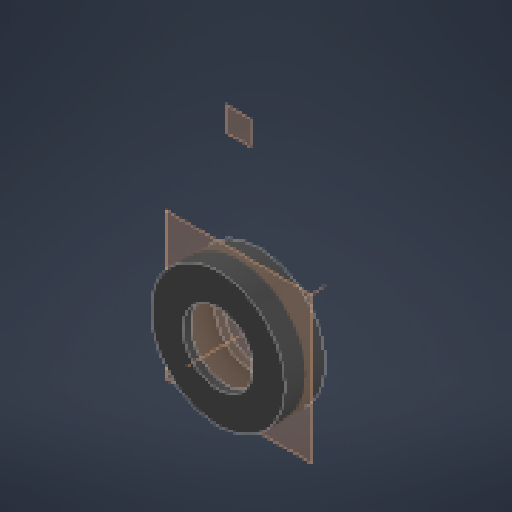
# Autodesk Inventor part: custom_bearing
Saved by Autodesk Inventor 2026.1 (Build 301233020, 233B)
## iProperties
Created: 2025-11-24
Part Number: custom_bearing
Material: 고무, 검은색
Document SubType Name: Modeling
Designer: jaewook
Density: 0.93 g/cm^3
Appearance: 고무 - 검은색
Author: jaewook
Autodesk Inventor part; units mm, degrees
ref_plane "YZ Plane" through (0, 0, 0) normal (1, 0, 0) x (0, 1, 0)
ref_plane "XZ Plane" through (0, 0, 0) normal (0, 1, 0) x (-1, 0, 0)
ref_plane "XY Plane" through (0, 0, 0) normal (0, 0, 1) x (1, 0, 0)
ref_plane "작업 평면1" through (0, -41, 8.5) normal (0, 0, 1) x (1, 0, 0)
sketch "스케치1" plane through (0, -41, 8.5) normal (0, 0, 1) x (1, 0, 0)
  circle A0 centre (0, -40.5) radius 15 projected
  circle A1 centre (0, -40.5) radius 5 projected
  circle A2 centre (0, -40.5) radius 14.8
  circle A3 centre (0, -40.5) radius 5.3
  circle A4 centre (0, -40.5) radius 13.1
  circle A5 centre (0, -40.5) radius 7
  point P0 (0, 41)
  dimension "d0" = 0.2
  dimension "d1" = 0.3
  dimension "d2" = 1.7
  dimension "d3" = 1.7
  constraints: 4 centre point
  measures "d0" radial gap between concentric circles of A0 A2
  measures "d1" radial gap between concentric circles of A1 A3
  measures "d2" radial gap between concentric circles of A3 A5
  measures "d3" radial gap between concentric circles of A2 A4
extrude "돌출1" add sketch "스케치1" along normal mid plane 9 contours A2
ref_plane "작업 평면2" through (0, -81.5, 8.5) normal (0, 0, 1) x (1, 0, 0)
sketch "스케치3" plane through (0, -81.5, 13) normal (0, 0, 1) x (1, 0, 0)
  circle A0 centre (0, 0) radius 13.1 projected
  circle A1 centre (0, 0) radius 7.8
  point P0 (0, 81.5)
  dimension "d11" = 5.3
  constraints: 1 centre point
  measures "d11" radial gap between concentric circles of A0 A1
extrude "돌출2" add sketch "스케치3" against normal up to surface (9 mm away)
sketch "스케치6" plane through (0, 0, 0) normal (1, 0, 0) x (0, 1, 0)
  line L0 (-96.3, 4) -> (-66.7, 4) projected
  line L1 (-66.7, 13) -> (-96.3, 13) projected
  line L2 (-66.7, 4) -> (-66.7, 13) projected
  line L3 (-96.3, 4) -> (-96.3, 13) projected
  circle A0 centre (-72.1, 8.5) radius 3.2
  line L4 (-81.5, -2.6) -> (-81.5, 15.6) projected
  line L5 (-68.9, 15.8649) -> (-68.9, 0.3346)
  circle A1 centre (-72.1, 8.5) radius 2.8 construction
  line L6 (-74.9, 15.3235) -> (-74.9, 0.5874) construction
  circle A2 centre (-71.7, 8.5) radius 2.8 construction
  line L7 (-74.5, 4.469) -> (-74.5, 12.0599) construction
  point P0 (0, 0)
  dimension "d19" = 6.4
  dimension "d21" = 4.5
  dimension "d22" = 29.6
  dimension "d23" = 2.2
  dimension "d25" = 5.6
  dimension "d26" = 5.6
  constraints: 6 end point, 4 tangent, 3 centre point, 3 vertical, 1 coincident, 1 horizontal alignment
  measures "d19" diameter of A0
  measures "d21" distance from line of L0 A0.centre
  measures "d22" distance of L1.start L1.end
  measures "d23" distance between parallel lines of L5 L2
  measures "d25" diameter of A1
  measures "d26" diameter of A2
revolve "회전2" cut sketch "스케치6" angle 360 about axis through (0, -81.5, 8.5) along (0, 0, 1) contours A0
